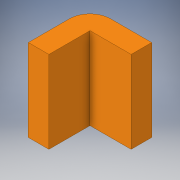
# Autodesk Inventor part: doorstop
Saved by Autodesk Inventor 2017 SP1 (Build 210196100, 196)
## iProperties
Created: 2018-09-12
Part Number: doorstop
Material: PC/ABS Plastic
Document SubType Name: Modeling
Designer: Delta
Density: 0.357273 g/cm^3
Appearance: Orange
Author: Delta
Autodesk Inventor part; units mm, degrees
ref_plane "YZ Plane" through (0, 0, 0) normal (1, 0, 0) x (0, 1, 0)
ref_plane "XZ Plane" through (0, 0, 0) normal (0, 1, 0) x (-1, 0, 0)
ref_plane "XY Plane" through (0, 0, 0) normal (0, 0, 1) x (1, 0, 0)
sketch "Sketch1" plane through (0, 0, 0) normal (0, 1, 0) x (-1, 0, 0)
  line L0 (0, 0) -> (38.1, 0)
  line L1 (38.1, 0) -> (38.1, 12.7)
  line L2 (38.1, 12.7) -> (0, 12.7)
  line L3 (0, 12.7) -> (0, 0)
  line L4 (38.1, 0) -> (25.4, 0)
  line L5 (25.4, 0) -> (25.4, 38.1)
  line L6 (25.4, 38.1) -> (38.1, 38.1)
  line L7 (38.1, 38.1) -> (38.1, 0)
  dimension "d0" = 38.1
  dimension "d1" = 12.7
  dimension "d2" = 38.1
  dimension "d3" = 12.7
  constraints: 16 end point, 4 parallel, 2 horizontal, 2 perpendicular
  measures "d0" distance of L2.end L1.end
  measures "d1" distance of L5.end L6.end
  measures "d2" distance of L4.end L5.end
  measures "d3" distance of L2.end L0.start
extrude "Extrusion1" add sketch "Sketch1" along normal blind 50.8
fillet "Fillet1" radius 12.7 1 edges at (-38.1, 25.4, 0)
equation "\"d3\" = d1"
body "Solid1"
